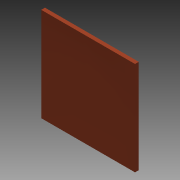
# Autodesk Inventor part: Copper Plate
Saved by Autodesk Inventor 2015 (Build 190159000, 159)
## iProperties
Created: 2015-10-12
Part Number: Copper Plate
Material: Copper
Document SubType Name: Modeling
Designer: Kyle
Density: 8.94 g/cm^3
Appearance: Copper - Satin
Author: Kyle
Autodesk Inventor part; units mm, degrees
ref_plane "YZ Plane" through (0, 0, 0) normal (1, 0, 0) x (0, 1, 0)
ref_plane "XZ Plane" through (0, 0, 0) normal (0, 1, 0) x (-1, 0, 0)
ref_plane "XY Plane" through (0, 0, 0) normal (0, 0, 1) x (1, 0, 0)
sketch "Sketch1" plane through (0, 0, 0) normal (0, 0, 1) x (1, 0, 0)
  line L0 (0, 0) -> (50.8, 0)
  line L1 (50.8, 0) -> (50.8, 50.8)
  line L2 (50.8, 50.8) -> (0, 50.8)
  line L3 (0, 50.8) -> (0, 0)
  dimension "d0" = 50.8
  dimension "d1" = 50.8
  constraints: 8 end point, 2 parallel, 1 horizontal, 1 perpendicular
  measures "d0" distance of L2.end L0.start
  measures "d1" distance of L0.start L0.end
extrude "Extrusion1" add sketch "Sketch1" along normal blind 2.032
body "Solid1"
